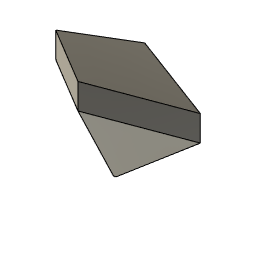
Final FFM PRINT v2 (Autodesk Fusion 360 design; units mm, degrees)
Autodesk Fusion 360 part; units mm, degrees
note: some values were not read from the file. Chosen so that the rebuilt part matches the saved one: which bodies a step acts on; which face or edge a step refers to.
sketch "Sketch1" plane through (0, 0, 0) normal (0, 0, 1) x (1, 0, 0)
  circle A0 centre (0, 0) radius 127
  dimension "d1" = 254
  constraint coincident A0.centre origin
  measures "d1" diameter of A0
extrude "Extrude1" add sketch "Sketch1" along normal blind 78.74 makes body 1
sketch "Sketch2" plane through (0, 0, 78.74) normal (0, 0, 1) x (-1, 0, 0)
  circle A0 centre (0, 0) radius 127
  circle A1 centre (0, 0) radius 127
  dimension "d4" = 254
  constraint coincident A0.centre A1.centre
  measures "d4" diameter of A1
extrude "Extrude2" add sketch "Sketch2" along normal blind 2.54 separate body makes body 2
move_body "Move1" bodies 2 to x (1, 0, 0) y (0, 1, 0) z (0, 0, 1) at (0, 0, -12.7)
extrude "Extrude3" cut 1 faces at (37.3597, -28.794, 66.04) along direction (0, 0, 1) blind 2.54 on bodies 2 bodies 1 2 makes body 3 at (-31.8845, 17.4247, 78.74)
move_body "Move2" bodies 3 to x (1, 0, 0) y (0, 1, 0) z (0, 0, 1) at (19.2726, -280.3292, 22.1586)
shell "Shell1" thickness 6.35 removed faces 1 at (-35.4503, -30.1567, 66.04) on bodies 1
chamfer "Chamfer1" distance 2.54 angle 45 1 edges at (-118.4056, -45.9252, 0) on bodies 1
chamfer "Chamfer2" distance 2.54 angle 45 1 edges at (-99.1329, -326.2543, 100.8986) on bodies 3
chamfer "Chamfer7" distance 1.27 angle 45 1 edges at (-112.4853, -43.6289, 6.35) on bodies 1
hole "Hole1" at (0, -127, 29.5911) direction (0, 1, 0) diameter 12.7 depth 261.62 tip angle 118 bodies 1
fillet "Fillet1" radius 1.27 1 edges at (6.35, -120.4828, 29.5911) on bodies 1
fillet "Fillet2" radius 1.27 1 edges at (6.35, 120.4828, 29.5911) on bodies 1
sketch "Sketch3" plane through (0, 0, 100.8986) normal (0, 0, 1) x (-1, 0, 0)
  circle A0 centre (-19.2726, 280.3292) radius 124.46
  line L0 (62.6341, 186.6191) -> (-101.1794, 186.6191)
  line L1 (62.6341, 374.0392) -> (-101.1794, 374.0392)
  line L2 (-101.1794, 186.6191) -> (-101.1794, 374.0392)
  line L3 (62.6341, 374.0392) -> (62.6341, 186.6191)
  constraint coincident A0 L0.start
  constraint coincident A0 L0.end
  constraint horizontal L0
  constraint coincident A0 L1.start
  constraint coincident A0 L1.end
  constraint parallel L0 L1
  constraint perpendicular L1 L2
extrude "Extrude4" cut sketch "Sketch3" against normal blind 2.54 contours L0 L1 L2 L3 bodies 3
sketch "Sketch4" plane through (0, 0, 100.8986) normal (0, 0, 1) x (-1, 0, 0)
  line L0 (62.6341, 374.0392) -> (62.6341, 186.6191)
  arc A0 (62.6341, 186.6191) -> (62.6341, 374.0392) centre (-19.2726, 280.3292) ccw
  line L1 (62.6341, 280.3292) -> (105.1874, 280.3292) construction
  line L2 (82.9532, 209.335) -> (84.0181, 349.7649) construction
  circle A1 centre (83.9107, 280.3292) radius 13.97
  dimension "d26" = 27.94
  constraint midpoint L0 L1.start
  constraint midpoint A0 L1.end
  constraint coincident A0 L2.start
  constraint coincident A0 L2.end
  constraint midpoint L1 A1.centre
  measures "d26" diameter of A1
extrude "Extrude5" add sketch "Sketch4" along normal blind 6.35 contours A1 bodies 2 3
extrude "Extrude6" cut 1 faces at (-82.8745, -269.4546, 107.2486) along direction (0, 0, -1) blind 2.54 on bodies 2 bodies 2
hole "Hole2" at (-83.9107, -280.3292, 104.7086) direction (0, 0, -1) diameter 11.43 depth 261.62 tip angle 118 bodies 2
fillet "Fillet3" radius 5.08 1 edges at (-70.8861, -285.3809, 104.7086) on bodies 2
chamfer "Chamfer8" distance 2.54 angle 45 1 edges at (-89.239, -282.3958, 90.7386) on bodies 2
sketch "Sketch5" plane through (0, 0, 0) normal (0, 0, -1) x (1, 0, 0)
  circle A0 centre (0, 0) radius 124.46
  line L0 (0, 0) -> (124.46, 0) construction
  line L1 (0, 0) -> (88.0065, 88.0065) construction
  line L2 (0, 0) -> (-87.8109, 87.8109) construction
  line L3 (0, 0) -> (-124.1834, 0) construction
  line L4 (0, 0) -> (88.0065, -88.0065) construction
  line L5 (0, 0) -> (-88.0065, -88.0065) construction
  line L6 (-88.0065, -88.0065) -> (88.0065, -88.0065) construction
  line L7 (-88.0065, -88.0065) -> (-87.8109, 87.8109) construction
  line L8 (-87.8109, 87.8109) -> (88.0065, 88.0065) construction
  line L9 (88.0065, 88.0065) -> (88.0065, -88.0065) construction
  line L10 (0, -124.46) -> (0, 124.46) construction
  line L11 (0, -107.0565) -> (-15.24, -107.0565) construction
  line L12 (-15.24, -107.0565) -> (-15.24, -40.64) construction
  line L13 (-15.24, -40.64) -> (0, -40.64) construction
  line L14 (0, -40.64) -> (0, -107.0565) construction
  line L15 (15.24, -40.64) -> (0, -40.64) construction
  line L16 (15.24, -107.0565) -> (15.24, -40.64) construction
  line L17 (0, -107.0565) -> (15.24, -107.0565) construction
  line L18 (0, -107.0565) -> (-15.24, -81.28)
  line L19 (-15.24, -81.28) -> (0, -40.64)
  line L20 (0, -40.64) -> (15.24, -81.28)
  line L21 (0, -107.0565) -> (15.24, -81.28)
  line L22 (-15.24, 107.0565) -> (-15.24, 40.64) construction
  line L23 (-15.24, 40.64) -> (0, 40.64) construction
  line L24 (0, 40.64) -> (15.24, 81.28)
  line L25 (0, 107.0565) -> (15.24, 107.0565) construction
  line L26 (0, 107.0565) -> (-15.24, 81.28)
  line L27 (0, 107.0565) -> (15.24, 81.28)
  line L28 (-15.24, 81.28) -> (0, 40.64)
  line L29 (0, 107.0565) -> (-15.24, 107.0565) construction
  line L30 (15.24, 107.0565) -> (15.24, 40.64) construction
  line L31 (15.24, 40.64) -> (0, 40.64) construction
  constraint horizontal L0
  constraint coincident A0.centre L0.start
  constraint horizontal L3
  constraint perpendicular L1 L4
  constraint horizontal L6
  constraint perpendicular L6 L9
  constraint coincident A0 L10.start
  constraint coincident A0 L10.end
  constraint vertical L10
  constraint horizontal L11
  constraint vertical L12
  constraint horizontal L13
  constraint vertical L14
  constraint coincident L10 L11.start
  constraint symmetric L10 L11.start L14.end
  constraint symmetric L10 L11.end L16.start
  constraint symmetric L10 L12.end L15.start
  constraint symmetric L10 L13.end L14.start
  constraint coincident L12 L18.end
  constraint coincident L16 L20.end
  constraint symmetric L3 L11.start L25.start
  constraint symmetric L3 L11.end L22.start
  constraint symmetric L3 L12.end L22.end
  constraint symmetric L3 L13.end L23.end
  constraint symmetric L3 L15.start L30.end
  constraint symmetric L3 L16.start L25.end
  constraint symmetric L3 L18.end L26.end
  constraint symmetric L3 L20.end L24.end
extrude "Extrude7" add 1 faces at (-35.8526, -17.2657, 6.35) along direction (0, 0, 1) blind 6.35 on bodies 1 bodies 1
fillet "Fillet4" radius 2.54 1 edges at (-111.3012, -43.1697, 12.7) on bodies 1
extrude "Extrude8" cut sketch "Sketch5" against normal blind 6.35 contours L24 L26 L27 L28 bodies 1
sketch "Sketch6" plane through (0, 0, 0) normal (0, 0, -1) x (1, 0, 0)
  line L0 (0, 40.64) -> (-15.24, 81.28)
  line L1 (-15.24, 81.28) -> (0, 107.0565)
  line L2 (0, 107.0565) -> (15.24, 81.28)
  line L3 (15.24, 81.28) -> (0, 40.64)
  circle A0 centre (0, 0) radius 124.46
  line L4 (-124.46, 0.0952) -> (124.4599, -0.1259) construction
  line L5 (-15.3844, -81.2835) -> (-0.1902, -107.0871)
  line L6 (-0.0722, -40.6707) -> (-15.3844, -81.2835)
  line L7 (-0.1902, -107.0871) -> (15.0956, -81.3377)
  line L8 (15.0956, -81.3377) -> (-0.0722, -40.6707)
  constraint coincident A0 L4.start
  constraint coincident A0 L4.end
  constraint symmetric L0.start L4 L6.start
  constraint symmetric L0.end L4 L5.start
  constraint symmetric L1.end L4 L5.end
  constraint symmetric L2.end L4 L7.end
extrude "Extrude9" cut sketch "Sketch6" against normal blind 6.35 contours L5 L6 L7 L8 bodies 1
sketch "Sketch7" plane through (0, 0, 0) normal (0, 0, -1) x (1, 0, 0)
  line L0 (-15.3844, -81.2835) -> (-0.0722, -40.6707)
  line L1 (-0.0722, -40.6707) -> (15.0956, -81.3377)
  line L2 (15.0956, -81.3377) -> (-0.1902, -107.0871)
  line L3 (-0.1902, -107.0871) -> (-15.3844, -81.2835)
  line L4 (0, 40.64) -> (-15.24, 81.28)
  line L5 (-15.24, 81.28) -> (0, 107.0565)
  line L6 (0, 107.0565) -> (15.24, 81.28)
  line L7 (15.24, 81.28) -> (0, 40.64)
  circle A0 centre (0, 0) radius 124.46
  line L8 (124.46, 0) -> (-124.46, 0) construction
  line L9 (0, -124.46) -> (0, 124.46) construction
  line L10 (0, 0) -> (-40.64, 0) construction
  line L11 (-124.46, 0) -> (-107.061, 0) construction
  line L12 (-107.061, 0) -> (-81.2847, 15.2441)
  line L13 (-107.061, 0) -> (-77.1144, 0) construction
  line L14 (-107.061, 0) -> (-81.2847, -15.2441)
  line L15 (-107.061, 0) -> (-77.1144, 0) construction
  line L16 (-81.2847, 15.2441) -> (-40.64, 0)
  line L17 (-40.64, 0) -> (-81.2847, -15.2441)
  line L18 (107.061, 0) -> (81.2847, -15.2441)
  line L19 (40.64, 0) -> (81.2847, -15.2441)
  line L20 (81.2847, 15.2441) -> (40.64, 0)
  line L21 (107.061, 0) -> (81.2847, 15.2441)
  dimension "d55" = 40.64
  dimension "d56" = 17.399
  dimension "d59" = 30.6
  dimension "d60" = 29.9466
  dimension "d61" = 30.6
  dimension "d62" = 29.9466
  constraint coincident A0 L8.start
  constraint coincident A0 L8.end
  constraint horizontal L8
  constraint coincident A0 L9.start
  constraint coincident A0 L9.end
  constraint perpendicular L8 L9
  constraint coincident A0.centre L10.start
  constraint perpendicular L9 L10
  constraint parallel L8 L11
  constraint horizontal L13
  constraint horizontal L15
  constraint symmetric L9 L10.end L19.start
  constraint symmetric L9 L11.end L18.start
  constraint symmetric L9 L12.end L20.start
  constraint symmetric L9 L14.end L18.end
  measures "d55" distance of A0.centre L10.end
  measures "d56" distance of L8.end L11.end
  measures "d59" angle of L12 L13
  measures "d60" distance of L11.end L12.end
  measures "d61" angle of L14 L15
  measures "d62" distance of L11.end L14.end
extrude "Extrude10" cut sketch "Sketch7" against normal blind 6.35 contours L12 L14 L16 L17 | L18 L19 L20 L21 bodies 1
ref_plane "WorkPlane1" through (-73.8505, 0, -19.05) normal (0, 0, -1) x (-1, 0, 0)
sketch "Sketch8" plane through (0, 0, 6.35) normal (0, 0, -1) x (1, 0, 0)
  line L0 (0, 107.0565) -> (-15.24, 81.28)
  line L1 (-15.24, 81.28) -> (0, 40.64)
  line L2 (0, 40.64) -> (15.24, 81.28)
  line L3 (15.24, 81.28) -> (0, 107.0565)
sketch "Sketch9" plane through (-73.8505, 0, -19.05) normal (0, 0, -1) x (1, 0, 0)
  line L0 (-33.02, 0) -> (-7.62, -15.24)
  line L1 (-7.62, -15.24) -> (33.02, 0)
  line L2 (33.02, 0) -> (-7.62, 15.24)
  line L3 (-7.62, 15.24) -> (-33.02, 0)
extrude "Extrude11" add sketch "Sketch9" along normal blind 38.1 separate body makes body 4
chamfer "Chamfer9" distance 13.716 angle 45 4 edges at (-61.1505, 7.62, -57.15) (-94.1705, 7.62, -57.15) (-94.1705, -7.62, -57.15) (-61.1505, -7.62, -57.15) on bodies 4
chamfer "Chamfer10" distance 19.05 angle 45 4 edges at (-94.1705, 7.62, -43.434) (-61.1505, 7.62, -43.434) (-61.1505, -7.62, -43.434) (-94.1705, -7.62, -43.434) on bodies 4
extrude "Extrude12" add 1 faces at (-67.9238, 0, -19.05) along direction (0, 0, 1) blind 6.35 on bodies 4 bodies 4
move_body "Move3" bodies 4 to x (1, 0, 0) y (0, 1, 0) z (0, 0, 1) at (-5.1195, -13.6519, -35.1998)
copy_body "CopyPasteBodies1" bodies 4 makes body 5
move_body "Move4" bodies 5 to x (1, 0, 0) y (0, 1, 0) z (0, 0, 1) at (68.58, 45.72, 0)
copy_body "CopyPasteBodies2" bodies 5 makes body 6
move_body "Move5" bodies 6 to x (1, 0, 0) y (0, 1, 0) z (0, 0, 1) at (-81.28, 50.8, 0)
copy_body "CopyPasteBodies3" bodies 4 makes body 7
move_body "Move6" bodies 7 to x (1, 0, 0) y (0, 1, 0) z (0, 0, 1) at (-119.38, 0, 0)
move_body "Move7" bodies 7 to x (1, 0, 0) y (0, 1, 0) z (0, 0, 1) at (-11.0022, -18.3369, 51.6264)
move_body "Move8" bodies 6 to x (1, 0, 0) y (0, 1, 0) z (0, 0, 1) at (-117.1164, -56.5866, -4.8601)
move_body "Move9" bodies 4 to x (1, 0, 0) y (0, 1, 0) z (0, 0, 1) at (-205.5638, -17.9447, -165.4966)
move_body "Move10" bodies 5 to x (1, 0, 0) y (0, 1, 0) z (0, 0, 1) at (-277.1726, -2.9686, -12.9774)
move_body "Move11" bodies 6 to x (1, 0, 0) y (0, 1, 0) z (0, 0, 1) at (-2.4065, 26.4238, 57.6909)
move_body "Move12" bodies 5 to x (1, 0, 0) y (0, 1, 0) z (0, 0, 1) at (-14.5538, 35.2634, 67.3759)
move_body "Move13" bodies 6 to x (1, 0, 0) y (0, 1, 0) z (0, 0, 1) at (5.1413, 11.5575, -30.3121)
move_body "Move14" bodies 7 to x (1, 0, 0) y (0, 1, 0) z (0, 0, 1) at (-0.5572, 40.6307, -0.2135)
move_body "Move15" bodies 5 to x (1, 0, 0) y (0, 1, 0) z (0, 0, 1) at (20.3066, 0.9987, 0)
move_body "Move16" bodies 4 to x (1, 0, 0) y (0, 1, 0) z (0, 0, 1) at (1.6645, 40.6133, 0)
move_body "Move17" bodies 6 to x (1, 0, 0) y (0, 1, 0) z (0, 0, 1) at (-3.9947, 0, 29.2948)
move_body "Move18" bodies 4 to x (1, 0, 0) y (0, 1, 0) z (0, 0, 1) at (1.5296, -108.5006, 220.1822)
move_body "Move19" bodies 4 to x (1, 0, 0) y (0, 1, 0) z (0, 0, 1) at (-0.3329, 109.1897, 0)
hole "Hole3" at (19.2726, -280.3292, 98.3586) direction (0, 0, -1) diameter 12.7 depth 152.4 tip angle 180 bodies 2
fillet "Fillet5" radius 12.7 1 edges at (13.3524, -282.6254, 90.7386) on bodies 2
chamfer "Chamfer11" distance 3.81 angle 45 2 edges at (-112.4853, 43.6289, 66.04) (-99.1329, -326.2543, 90.7386) on bodies 1 2
extrude "Extrude14" add 1 faces at (19.2726, -215.7391, 98.3586) along direction (0, 0, 1) blind 2.54 on bodies 2 bodies 2
extrude "Extrude15" cut 1 faces at (-80.4734, -287.4669, 104.7086) along direction (0, 0, -1) blind 2.54 on bodies 2 bodies 2
delete_face "DeleteFace1" 3 faces at (-74.7119, -269.9056, 101.1372) (-87.6334, -288.5795, 103.0153) (-80.4734, -287.4669, 102.1686) on bodies 2
hidden bodies 1 2 4 5 6
named bodies: "Body", "Lid", "Spike 2", "Spike 3", "Spike 4", "Spike 1"
